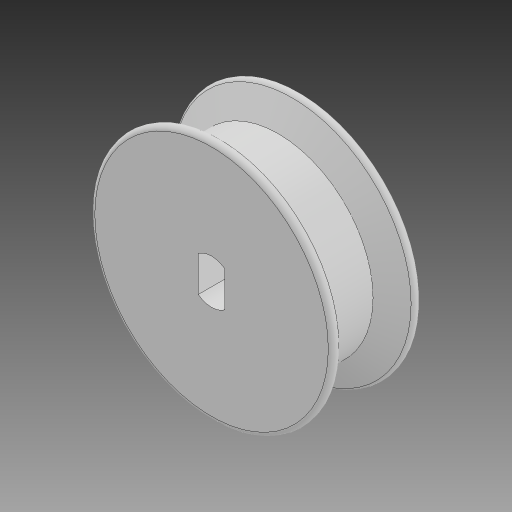
# Autodesk Inventor part: rub-ring
Saved by Autodesk Inventor 2023 (Build 270158000, 158)
## iProperties
Created: 2024-02-02
Part Number: rub-ring
Material: Všeobecné
Document SubType Name: Modeling
Designer: matej
Mass: 4.15328 g
Surface Area: 22.3088 cm^2
Volume: 4.15328 cm^3
Density: 1 g/cm^3
Appearance: Výchozí
Author: matej
Autodesk Inventor part; units mm, degrees
ref_plane "YZ Plane" through (0, 0, 0) normal (1, 0, 0) x (0, 1, 0)
ref_plane "XZ Plane" through (0, 0, 0) normal (0, 1, 0) x (-1, 0, 0)
ref_plane "XY Plane" through (0, 0, 0) normal (0, 0, 1) x (1, 0, 0)
sketch "Náčrt1" plane through (0, 0, 0) normal (0, 0, 1) x (1, 0, 0)
  circle A0 centre (0, 0) radius 2.5
  line L0 (-1.5, -2.5) -> (1.5, -2.5)
  line L1 (1.5, -2.5) -> (1.5, 2.5)
  line L2 (1.5, 2.5) -> (-1.5, 2.5)
  line L3 (-1.5, 2.5) -> (-1.5, -2.5)
  line L4 (-1.5, -2.5) -> (1.5, 2.5) construction
  line L5 (1.5, -2.5) -> (-1.5, 2.5) construction
  circle A1 centre (0, 0) radius 15
  point P0 (-1.5, -2)
  point P1 (-1.5, 2)
  point P2 (1.5, 2)
  point P3 (1.5, -2)
  dimension "d0" = 5
  dimension "d1" = 3
  dimension "d2" = 5
  dimension "d3" = 30
  constraints: 12 end point, 2 centre point, 2 coincident, 2 midpoint, 2 parallel, 1 horizontal, 1 perpendicular
  measures "d0" diameter of A0
  measures "d1" distance of L2.end L1.end
  measures "d2" distance of L1.end L0.end
  measures "d3" diameter of A1
extrude "Vysunutí1" add sketch "Náčrt1" along normal blind 10 contours A0 L1 | A0 L2 L1 | L1 L0 A0 | A0 L3 L2 | L0 L3 A0 | L3 A0 | A1
sketch "Náčrt2" plane through (0, 0, 0) normal (1, 0, 0) x (0, 1, 0)
  line L0 (15, 0) -> (-15, 0) projected
  line L1 (15, 10) -> (-15, 10) projected
  line L2 (15, 0) -> (15, 10)
  line L3 (15, 10) -> (10.6699, 7.5)
  line L4 (15, 0) -> (10.6699, 2.5)
  line L5 (10.6699, 2.5) -> (10.6699, 7.5)
  line L6 (0, -2) -> (0, 12) projected
  point P0 (0, 0)
  dimension "d6" = 5
  dimension "d7" = 60
  dimension "d8" = 60
  dimension "d9" = 5
  constraints: 8 end point, 1 vertical
  measures "d6" distance of L1.start L3.end
  measures "d7" angle of L3 L2
  measures "d8" angle of L2 L4
  measures "d9" distance of L4.end L3.end
revolve "Rotace1" cut sketch "Náčrt2" angle 360 about axis through (0, 0, -10) along (0, 0, 1) contours L4 L5 L3 L2
fillet "Zaoblení1" radius 0.5 2 edges at (0, -15, 0) (0, -15, 10)
equation "\"d8\" = d7"
